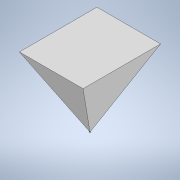
# Autodesk Inventor part: FieldofView
Saved by Autodesk Inventor 2020 (Build 240168000, 168)
## iProperties
Created: 2019-11-08
Part Number: FieldofView
Material: Generic
Document SubType Name: Modeling
Designer: nicoc
Density: 1 g/cm^3
Appearance: Default
Author: nicoc
Autodesk Inventor part; units mm, degrees
ref_plane "YZ Plane" through (0, 0, 0) normal (1, 0, 0) x (0, 1, 0)
ref_plane "XZ Plane" through (0, 0, 0) normal (0, 1, 0) x (-1, 0, 0)
ref_plane "XY Plane" through (0, 0, 0) normal (0, 0, 1) x (1, 0, 0)
sketch "Sketch1" plane through (0, 0, 0) normal (0, 1, 0) x (-1, 0, 0)
  line L0 (0, 0) -> (550, 0)
  line L1 (550, 0) -> (550, -670)
  line L2 (550, -670) -> (0, -670)
  line L3 (0, -670) -> (0, 0)
  dimension "d0" = 670
  dimension "d1" = 550
  constraints: 8 end point, 2 parallel, 1 horizontal, 1 perpendicular
  measures "d0" distance between parallel lines of L2 L0
  measures "d1" distance between parallel lines of L1 L3
extrude "Extrusion1" add sketch "Sketch1" along normal blind 630
sketch "Sketch5" plane through (0, 0, 0) normal (1, 0, 0) x (0, 0, -1)
  line L0 (0, 630) -> (0, 0)
  line L1 (0, 0) -> (335, 0)
  line L2 (0, 0) -> (670, 0) projected
  line L3 (0, 630) -> (335, 0)
  constraints: 6 end point, 1 midpoint, 1 vertical
extrude "Extrusion2" cut sketch "Sketch5" against normal through all
sketch "Sketch6" plane through (0, 0, -670) normal (1, 0, 0) x (0, 0, -1)
  line L0 (-670, 630) -> (-335, 0) projected
  line L1 (-335, 0) -> (0, 630)
  line L2 (0, 630) -> (0, 0)
  line L3 (0, 0) -> (-335, 0)
  point P0 (-670, 0)
  constraints: 6 end point, 1 vertical
extrude "Extrusion3" cut sketch "Sketch6" against normal through all
sketch "Sketch8" plane through (0, 0, 0) normal (0, 0, 1) x (1, 0, 0)
  line L0 (-550, 630) -> (0, 630) projected
  line L1 (-550, 0) -> (-550, 630) projected
  line L2 (-550, 630) -> (-550, 0)
  line L3 (-550, 0) -> (-275, 0)
  line L4 (-275, 0) -> (-550, 630)
  point P0 (0, 0)
  dimension "d8" = 275
  constraints: 6 end point, 1 collinear, 1 perpendicular
  measures "d8" distance from line of L3.end L1
extrude "Extrusion4" cut sketch "Sketch8" against normal through all
sketch "Sketch9" plane through (0, 0, 0) normal (0, 0, 1) x (1, 0, 0)
  line L0 (0, 0) -> (-275, 0) projected
  line L1 (-275, 0) -> (0, 630)
  line L2 (0, 630) -> (0, 0)
  constraints: 4 end point, 1 vertical
extrude "Extrusion5" cut sketch "Sketch9" against normal through all
sketch "Sketch10" plane through (0, 0, 0) normal (0, 1, 0) x (-1, 0, 0)
  line L0 (270, -330) -> (280, -330)
  line L1 (280, -330) -> (280, -340)
  line L2 (280, -340) -> (270, -340)
  line L3 (270, -340) -> (270, -330)
  line L4 (550, 0) -> (0, 0) projected
  line L5 (0, 0) -> (0, -670) projected
  dimension "d13" = 10
  dimension "d14" = 10
  dimension "d15" = 330
  dimension "d16" = 270
  constraints: 8 end point, 2 parallel, 1 horizontal, 1 perpendicular
  measures "d13" distance between parallel lines of L2 L0
  measures "d14" distance between parallel lines of L3 L1
  measures "d15" distance between parallel lines of L4 L0
  measures "d16" distance between parallel lines of L5 L3
extrude "Extrusion6" add sketch "Sketch10" along normal blind 0.1
body "Solid1"
